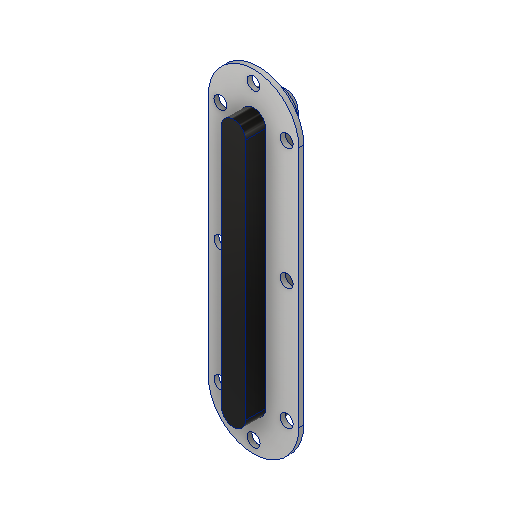
# Autodesk Inventor part: ASSEMBLY_Regolith_level_sensor
Saved by Autodesk Inventor 2025 (Build 290162010, 162A)
## iProperties
Created: 2018-09-12
Part Number: ASSEMBLY_Regolith_level_sensor
Material: Aluminum 6061
Document SubType Name: Modeling
Designer: Andrzej
Density: 2.7 g/cm^3
Appearance: Aluminum - Flat
Mass: 2.82067 g
Surface Area: 13.4574 cm^2
Volume: 1.04469 cm^3
Author: Andrzej
Autodesk Inventor part; units mm, degrees
ref_plane "YZ Plane" through (0, 0, 0) normal (1, 0, 0) x (0, 1, 0)
ref_plane "XZ Plane" through (0, 0, 0) normal (0, 1, 0) x (-1, 0, 0)
ref_plane "XY Plane" through (0, 0, 0) normal (0, 0, 1) x (1, 0, 0)
sketch "Sketch1" plane through (0, 0, 0) normal (0, 0, 1) x (1, 0, 0)
  line L0 (0, -7.3524) -> (0, 22.6476) construction
  line L1 (1.5, -7.3524) -> (1.5, 22.6476)
  line L2 (-1.5, 22.6476) -> (-1.5, -7.3524)
  arc A0 (-1.5, -7.3524) -> (1.5, -7.3524) centre (0, -7.3524) ccw
  arc A1 (1.5, 22.6476) -> (-1.5, 22.6476) centre (0, 22.6476) ccw
  line L3 (-2.5, -7.3524) -> (-2.5, 22.6476)
  arc A2 (2.5, 22.6476) -> (-2.5, 22.6476) centre (0, 22.6476) ccw
  line L4 (2.5, 22.6476) -> (2.5, -7.3524)
  arc A3 (-2.5, -7.3524) -> (2.5, -7.3524) centre (0, -7.3524) ccw
  line L5 (-5.6, 22.6476) -> (-5.6, -7.3524)
  arc A4 (-5.6, -7.3524) -> (5.6, -7.3524) centre (0, -7.3524) ccw
  line L6 (5.6, -7.3524) -> (5.6, 22.6476)
  arc A5 (5.6, 22.6476) -> (-5.6, 22.6476) centre (0, 22.6476) ccw
  line L7 (-4.1, 22.6476) -> (-4.1, -7.3524)
  arc A6 (-4.1, -7.3524) -> (4.1, -7.3524) centre (0, -7.3524) ccw
  line L8 (4.1, -7.3524) -> (4.1, 22.6476)
  arc A7 (4.1, 22.6476) -> (-4.1, 22.6476) centre (0, 22.6476) ccw
  point P0 (0, 0)
  point P1 (0, 7.6476)
  point P2 (0, 26.7476)
  point P3 (0, -11.4524)
  point P4 (-4.1, 7.6476)
  point P5 (-4.1, 22.6476)
  point P6 (4.1, 7.6476)
  point P7 (-4.1, 7.6476)
  dimension "d0" = 30
  dimension "d1" = 3
  dimension "d2" = 1
  dimension "d3" = 3.1
  dimension "d10" = 1.6
  dimension "d16" = 15
  constraints: 20 end point, 18 point on circle, 8 centre point, 4 parallel, 4 tangent, 3 coincident, 3 midpoint, 2 vertical, 1 horizontal alignment, 11 other
  measures "d0" distance of L0.start L0.end
  measures "d1" diameter of A1
  measures "d2" distance between parallel lines of L2 L3
  measures "d3" distance between parallel lines of L3 L5
  measures "d10" distance between parallel lines of L3 L7
  measures "d16" distance of point (-4.1, -7.352) point (-4.1, 7.648)
extrude "Extrusion1" add sketch "Sketch1" along normal blind 2.5 contours A0 L2 A1 L1
extrude "Extrusion2" add sketch "Sketch1" against normal blind 0.6 contours A5 L6 A4 L5 | A7 L8 A6 L7
extrude "Extrusion3" add sketch "Sketch1" against normal blind 4 contours A0 L2 A1 L1 | L3 A2 L4 A3
hole "Hole1" at (0, 26.7476, 0) at (0, -11.4524, 0) at (-4.1, -7.3524, 0) at (-4.1, 7.6476, 0) at (-4.1, 22.6476, 0) at (4.1, -7.3524, 0) at (4.1, 7.6476, 0) at (4.1, 22.6476, 0) direction (0, 0, -1) diameter 1.6 end through all both
chamfer "Chamfer1" distance 1 angle 45 4 edges at (0, -9.8524, -4) (-2.5, 7.6476, -4) (0, 25.1476, -4) (2.5, 7.6476, -4)
sketch "Sketch2" plane through (-2.5, -7.3524, -0.6) normal (-1, 0, 0) x (0, 0, 1)
  line L0 (-2.4, 0) -> (-2.4, 30) projected
  line L1 (0, 0) -> (-2.4, 0) projected
  line L2 (0, 30) -> (0, 0) projected
  line L3 (0, 30) -> (-2.4, 30) projected
  line L4 (-2.4, 30) -> (-2.4, 0) projected
  line L5 (-2.4, 1.2) -> (-2.4, 3.2) construction
  line L6 (-1.9, 1.2) -> (-1.9, 3.2)
  line L7 (-2.9, 3.2) -> (-2.9, 1.2)
  arc A0 (-2.9, 1.2) -> (-1.9, 1.2) centre (-2.4, 1.2) ccw
  arc A1 (-1.9, 3.2) -> (-2.9, 3.2) centre (-2.4, 3.2) ccw
  line L8 (-1.4, 1.2) -> (-1.4, 3.2)
  arc A2 (-1.4, 3.2) -> (-3.4, 3.2) centre (-2.4, 3.2) ccw
  line L9 (-3.4, 3.2) -> (-3.4, 1.2)
  arc A3 (-3.4, 1.2) -> (-1.4, 1.2) centre (-2.4, 1.2) ccw
  circle A4 centre (-2.4, 1.2) radius 0.5
  circle A5 centre (-2.4, 3.2) radius 0.5
  circle A6 centre (-2.4, 2.2) radius 0.5
  point P0 (0.6, 7.3524)
  dimension "d31" = 2
  dimension "d32" = 1
  dimension "d33" = 1.2
  dimension "d34" = 0.5
  constraints: 12 end point, 8 point on circle, 5 centre point, 5 tangent, 3 coincident, 2 horizontal alignment, 2 parallel, 2 point on line, 1 midpoint, 7 other
  measures "d31" distance of L5.start L5.end
  measures "d32" diameter of A1
  measures "d33" distance from line of L1 L5.start
  measures "d34" radial gap between concentric circles of A0 A3
extrude "Extrusion5" add sketch "Sketch2" against normal blind 1 contours A3 L9 A2 L0 A1 L7 A0 | L0 A0 L6 A1 A2 L8 A3
extrude "Extrusion6" add sketch "Sketch2" along normal mid plane 8 contours A0 A4 L0 | L0 A4 A0 | A6 L0 | L0 A6 | A5 A1 L0 | L0 A1 A5
body "Solid1"
